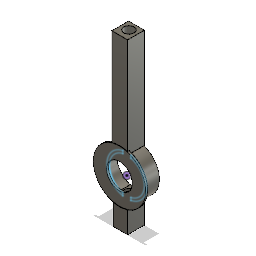
DropperCasing v8 (Autodesk Fusion 360 design; units mm, degrees)
Autodesk Fusion 360 part; units mm, degrees
sketch "dropper" plane through (0, 0, 0) normal (0, 0, 1) x (1, 0, 0)
  arc A0 (-2.425, 10.2161) -> (-2.425, -10.2161) centre (0, 0) ccw
  arc A1 (2.425, -10.2161) -> (2.425, 10.2161) centre (0, 0) ccw
  arc A2 (-2.425, 11.7524) -> (-2.425, -11.7524) centre (0, 0) ccw
  arc A3 (2.425, -11.7524) -> (2.425, 11.7524) centre (0, 0) ccw
  line L0 (-2.425, 11.7524) -> (-2.425, 10.2161)
  line L1 (2.425, 11.7524) -> (2.425, 10.2161)
  line L2 (-2.425, -10.2161) -> (-2.425, -11.7524)
  line L3 (2.425, -10.2161) -> (2.425, -11.7524)
  constraint coincident A0.centre A1.centre
  constraint concentric A0 A1
  constraint concentric A2 A3
extrude "Extrude1" add sketch "dropper" along normal blind 3 contours A1 A3 L1 L3 makes body 1
extrude "Extrude2" add sketch "dropper" along normal blind 3 separate body contours A0 A2 L0 L2 makes body 2
extrude "Extrude3" add sketch "dropper" against normal blind 3 contours A1 A3 L1 L3 bodies 1
extrude "Extrude4" add sketch "dropper" against normal blind 3 contours A0 A2 L0 L2 bodies 2
combine "Combine1" operation add target body 1 tool bodies 2 makes body 3 at (-2.9858, -11.6226, 1)
sketch "Sketch4" plane through (0, 0, 3) normal (0, 0, 1) x (1, 0, 0)
  line L0 (2.425, -10.2161) -> (2.425, -11.7524)
  arc A0 (2.425, -11.7524) -> (2.425, 11.7524) centre (0, 0) ccw
  line L1 (2.425, 11.7524) -> (2.425, 10.2161)
  arc A1 (2.425, -10.2161) -> (2.425, 10.2161) centre (0, 0) ccw
  circle A2 centre (0, 0) radius 13.7425
  constraint coincident A0.centre A1.centre
extrude "Extrude6" add sketch "Sketch4" along normal blind 1 bodies 3 1
extrude "Extrude7" add 1 faces at (11.4793, 0, 3) along direction (0, 0, 1) blind 1 on bodies 3 bodies 3
copy_body "CopyPasteBodies3" bodies 3 makes body 4
move_body "Move8" bodies 4 to x (1, 0, 0) y (0, 1, 0) z (0, 0, 1) at (-31, 0, 0)
scale "Scale5" factor 1.15 about (2.425, -10.2161, 3) bodies 3
scale "Scale6" factor 1.25 about (-28.575, 10.2161, 3) bodies 4
move_body "Move9" bodies 4 to x (1, 0, 0) y (0, 1, 0) z (0, 0, 1) at (-5, 0, 0)
sketch "Sketch5" plane through (0, 0, 4.25) normal (0, 0, 1) x (1, 0, 0)
  circle A0 centre (-36.6063, -2.554) radius 17.1781
  circle A1 centre (-36.6063, -2.554) radius 8.7958
  constraint concentric A0 A1
sketch "Sketch6" plane through (0, 0, 4.15) normal (0, 0, 1) x (1, 0, 0)
  circle A0 centre (-0.3637, 1.5324) radius 15.8038
  circle A1 centre (-0.3637, 1.5324) radius 7.6718
  constraint concentric A0 A1
sketch "Sketch7" plane through (0, 0, 4.15) normal (0, 0, 1) x (1, 0, 0)
extrude "Extrude8" cut sketch "Sketch6" against normal blind 1 contours A1 bodies 3
extrude "Extrude9" cut 1 faces at (-2.0582, 1.9254, 3.15) along direction (0, 0, -1) blind 1 on bodies 3 bodies 3
extrude "Extrude10" cut sketch "Sketch5" against normal blind 2 contours A1 bodies 4
extrude "Extrude11" add 1 faces at (12.8374, 1.5324, -3.9) along direction (0, 0, -1) blind 2.3 on bodies 3 bodies 3
extrude "Extrude12" add 1 faces at (-13.5649, 1.5324, -3.9) along direction (0, 0, -1) blind 2.3 on bodies 3 bodies 3
delete_body "RemoveBody1" bodies 4
extrude "Extrude13" cut 1 faces at (2.425, 14.4588, -3.1333) along direction (1, 0, 0) blind 1 on bodies 3 bodies 3
extrude "Extrude14" cut 1 faces at (-3.1525, 14.4588, -3.1333) along direction (-1, 0, 0) blind 1 on bodies 3 bodies 3
extrude "Extrude15" cut 2 faces at (-3.4858, 13.281, -3.1333) (2.7583, 13.281, -0.0667) along direction (0, -1, 0) blind 100 on bodies 3 bodies 3
extrude "Extrude16" add 1 faces at (3.425, 14.2006, -3.1333) along direction (-1, 0, 0) blind 7.578 on bodies 3 bodies 3
extrude "Extrude17" add 1 faces at (3.425, -10.5343, -0.0667) along direction (-1, 0, 0) blind 7.577 on bodies 3 bodies 3
extrude "Extrude18" add 1 faces at (-1.627, 14.8021, -3.1333) along direction (0, 1, 0) blind 100 on bodies 3 bodies 3
extrude "Extrude19" add 1 faces at (-1.6263, -11.7373, -3.1333) along direction (0, -1, 0) blind 20 on bodies 3 bodies 3
extrude "Extrude20" cut 1 faces at (-1.627, 114.8021, -3.1333) along direction (0, -1, 0) blind 20 on bodies 3 bodies 3
extrude "Extrude21" cut 1 faces at (-1.6263, -31.7373, -3.1333) along direction (0, 1, 0) blind 5 on bodies 3 bodies 3
sketch "Sketch8" plane through (0, -26.7373, 0) normal (0, -1, 0) x (1, 0, 0)
  line L0 (3.425, -6.2) -> (3.425, 3)
  line L1 (3.425, 3) -> (-4.152, 3)
  line L2 (-4.152, 3) -> (-4.152, -6.2)
  line L3 (-4.152, -6.2) -> (3.425, -6.2)
  line L4 (3.425, -6.2) -> (-4.152, 3) construction
  line L5 (3.425, 3) -> (-4.152, -6.2) construction
  circle A0 centre (-0.3635, -1.6) radius 3.1
  dimension "d52" = 6.2
  constraint coincident L0.start L3.end
  constraint coincident L1.end L2.start
  constraint coincident L0.end L1.start
  constraint coincident L2.end L3.start
  constraint midpoint L4 A0.centre
  measures "d52" diameter of A0
extrude "Extrude22" cut sketch "Sketch8" against normal blind 200 contours A0 bodies 3
extrude "Extrude23" add 1 faces at (-4.153, 42.1598, -3.1333) along direction (-1, 0, 0) blind 1 on bodies 3 bodies 3
extrude "Extrude24" add 1 faces at (3.425, 42.1599, -3.1333) along direction (1, 0, 0) blind 1 on bodies 3 bodies 3
extrude "Extrude25" add 1 faces at (-0.0398, 68.9702, 3) along direction (0, 0, 1) blind 1 on bodies 3 bodies 3
extrude "Extrude26" add 1 faces at (-0.3635, -22.582, 3) along direction (0, 0, 1) blind 1 on bodies 3 bodies 3
extrude "Extrude27" add 1 faces at (3.425, -17.4284, -3.1333) along direction (1, 0, 0) blind 1 on bodies 3 bodies 3
extrude "Extrude28" cut 1 faces at (-4.152, -16.8269, -3.1333) along direction (-1, 0, 0) blind 1 on bodies 3 bodies 3
extrude "Extrude29" cut 1 faces at (-0.4411, 94.8021, 3.1638) along direction (0, -1, 0) blind 20 on bodies 3 bodies 3
move_body "Move1" [suppressed]
ref_plane "WorkPlane1" through (2, 12, -2.6079) normal (0, 1, 0) x (1, 0, 0)
move_body "Move2" [suppressed]
move_body "Move3" [suppressed]
sketch "Sketch3" plane through (0, 0, -3) normal (0, 0, -1) x (-1, 0, 0)
  line L0 (-3.425, -11.7524) -> (-3.425, -10.2161)
  arc A0 (-3.425, 10.2161) -> (-3.425, -10.2161) centre (-1, 0) ccw
  line L1 (-3.425, 10.2161) -> (-3.425, 11.7524)
  arc A1 (-3.425, 11.7524) -> (-3.425, -11.7524) centre (-1, 0) ccw
  circle A2 centre (0, 0) radius 15.4529
  constraint coincident A2.centre origin
extrude "Extrude5" [suppressed]
copy_body "CopyPasteBodies1" [suppressed]
move_body "Move4" [suppressed]
scale "Scale2" [suppressed]
move_body "Move7" [suppressed]
scale "Scale4" [suppressed]
scale "Scale1" [suppressed]
